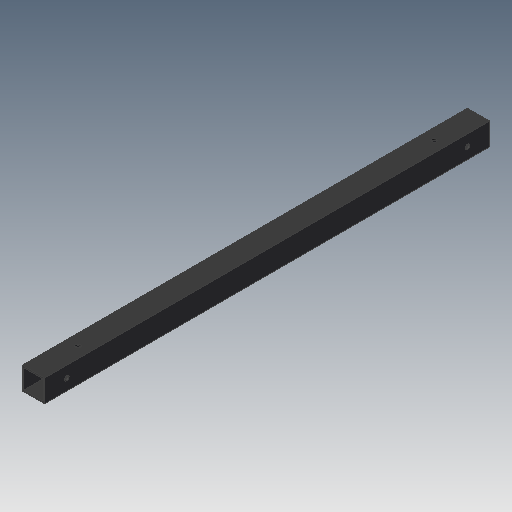
# Autodesk Inventor part: 回路角柱
Saved by Autodesk Inventor 2019.4 (Build 234330000, 330)
## iProperties
Created: 2018-06-23
Part Number: 回路角柱
Material: 一般
Document SubType Name: Modeling
Designer: AzLIer
Density: 1 g/cm^3
Appearance: 既定
Mass: 16.7357 g
Surface Area: 336.637 cm^2
Volume: 16.7357 cm^3
Author: AzLIer
Autodesk Inventor part; units mm, degrees
ref_plane "YZ Plane" through (0, 0, 0) normal (1, 0, 0) x (0, 1, 0)
ref_plane "XZ Plane" through (0, 0, 0) normal (0, 1, 0) x (-1, 0, 0)
ref_plane "XY Plane" through (0, 0, 0) normal (0, 0, 1) x (1, 0, 0)
sketch "スケッチ1" plane through (0, 0, 0) normal (0, 0, 1) x (1, 0, 0)
  line L0 (-7.5, 7.5) -> (7.5, 7.5)
  line L1 (7.5, 7.5) -> (7.5, -7.5)
  line L2 (7.5, -7.5) -> (-7.5, -7.5)
  line L3 (-7.5, -7.5) -> (-7.5, 7.5)
  line L4 (-7.5, 7.5) -> (7.5, -7.5) construction
  line L5 (7.5, 7.5) -> (-7.5, -7.5) construction
  line L6 (-6.5, -6.5) -> (6.5, -6.5)
  line L7 (6.5, -6.5) -> (6.5, 6.5)
  line L8 (6.5, 6.5) -> (-6.5, 6.5)
  line L9 (-6.5, 6.5) -> (-6.5, -6.5)
  point P0 (0, 0)
  dimension "d0" = 15
  dimension "d1" = 15
  constraints: 20 end point, 2 midpoint, 2 parallel, 1 horizontal, 1 perpendicular
  measures "d0" distance of L1.end L2.end
  measures "d1" distance of L0.end L1.end
extrude "押し出し1" add sketch "スケッチ1" along normal mid plane 300
sketch "スケッチ2" plane through (-7.5, -7.5, 150) normal (0, -1, 0) x (1, 0, 0)
  line L0 (7.5, -270) -> (7.5, -30)
  point P0 (7.5, -150)
  point P1 (7.5, -150)
  dimension "d4" = 240
  constraints: 2 end point, 1 coincident, 1 midpoint, 1 vertical
  measures "d4" distance of L0.start L0.end
hole "穴1" at (0, -7.5, 120) at (0, -7.5, -120) direction (0, 1, 0) diameter 3.2 end through all
sketch "スケッチ3" plane through (-7.5, -7.5, 150) normal (-1, 0, 0) x (0, 0, 1)
  line L0 (-285, 7.5) -> (-15, 7.5)
  point P0 (-150, 7.5)
  point P1 (-150, 7.5)
  dimension "d12" = 270
  constraints: 3 coincident, 2 end point, 1 horizontal, 1 midpoint
  measures "d12" distance of L0.start L0.end
hole "穴2" at (-7.5, 0, -135) at (-7.5, 0, 135) direction (1, 0, 0) diameter 3.2 end through all
